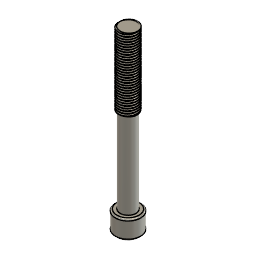
Tige_filetéeM5_5 (Autodesk Fusion 360 design; units mm, degrees)
part number: 2026-08-19-09-42-57-255
Autodesk Fusion 360 part; units mm, degrees
sketch "Esquisse1" plane through (0, 0, 0) normal (0, 1, 0) x (1, 0, 0)
  circle A0 centre (0, 0) radius 2.5
  circle A1 centre (0, 0) radius 4
  dimension "d1" = 5
  dimension "d4" = 8
  constraint coincident A0.centre A1.centre
  constraint concentric A0 A1
  measures "d1" diameter of A0
  measures "d4" diameter of A1
extrude "Extrusion1" add sketch "Esquisse1" along normal blind 27 contours A0 makes body 1
extrude "Extrusion2" add sketch "Esquisse1" against normal blind 6 separate body contours A0 | A1 makes body 2
extrude "Extrusion3" add 1 faces at (-0.8863, 27, -0.2321) along direction (0, 1, 0) blind 23 separate body on bodies 1 makes body 3
thread "Filetage1" "ISO Metric profile 6.0 M6x0.7 M6x0.7 6g" major diameter 5.908 minor diameter 5.1087 pitch 0.7 angle 60 modelled right hand crest width 0.1005 on face at (2.4969, 42.3333, 0.1246) crest through (2.954, 26.825, 0) on bodies 3
sketch "Esquisse2" plane through (0, -6, 0) normal (0, -1, 0) x (1, 0, 0)
  circle A0 centre (0, 0) radius 4
  line L0 (-2.2451, 0.5413) -> (-1.5913, -1.6736)
  line L1 (-1.5913, -1.6736) -> (0.6537, -2.2149)
  line L2 (0.6537, -2.2149) -> (2.2451, -0.5413)
  line L3 (2.2451, -0.5413) -> (1.5913, 1.6736)
  line L4 (1.5913, 1.6736) -> (-0.6537, 2.2149)
  line L5 (-0.6537, 2.2149) -> (-2.2451, 0.5413)
  dimension "d11" = 4
  constraint coincident A0.centre origin
  measures "d11" distance of L1 L4
extrude "Extrusion4" cut sketch "Esquisse2" against normal blind 4 contours L0 L1 L2 L3 L4 L5 bodies 2
fillet "Congé3" radius 1.5 6 edges at (0.4688, -2, 1.9443) (1.9182, -2, 0.5662) (-1.4494, -2, 1.3781) (-1.9182, -2, -0.5662) (1.4494, -2, -1.3781) (-0.4688, -2, -1.9443) on bodies 2
fillet "Congé2" radius 0.5 2 edges at (-3.7293, -6, -1.4465) (-3.7293, 0, 1.4465) on bodies 2
